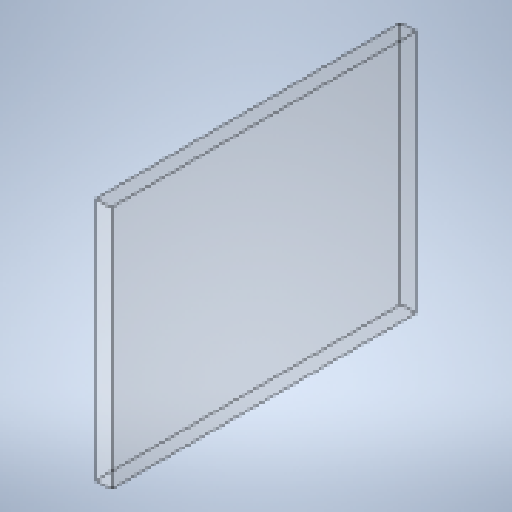
# Autodesk Inventor part: Cover
Saved by Autodesk Inventor 2023.2 (Build 272271000, 271)
## iProperties
Created: 2024-03-02
Part Number: Cover
Material: Polycarbonate, Clear
Document SubType Name: Modeling
Designer: Nathan Cai
Density: 1.2 g/cm^3
Appearance: Polycarbonate - Clear
Author: Nathan Cai
Autodesk Inventor part; units mm, degrees
ref_plane "YZ Plane" through (0, 0, 0) normal (1, 0, 0) x (0, 1, 0)
ref_plane "XZ Plane" through (0, 0, 0) normal (0, 1, 0) x (-1, 0, 0)
ref_plane "XY Plane" through (0, 0, 0) normal (0, 0, 1) x (1, 0, 0)
sketch "Sketch1" plane through (0, 0, 0) normal (1, 0, 0) x (0, 1, 0)
  line L0 (-22.225, -31.75) -> (22.225, -31.75)
  line L1 (22.225, -31.75) -> (22.225, 31.75)
  line L2 (22.225, 31.75) -> (-22.225, 31.75)
  line L3 (-22.225, 31.75) -> (-22.225, -31.75)
  line L4 (-22.225, -31.75) -> (22.225, 31.75) construction
  line L5 (22.225, -31.75) -> (-22.225, 31.75) construction
  point P0 (0, 0)
  dimension "d0" = 44.45
  dimension "d1" = 63.5
  constraints: 12 end point, 2 midpoint, 2 parallel, 1 horizontal, 1 perpendicular
  measures "d0" distance of L2.end L1.end
  measures "d1" distance of L1.end L0.end
extrude "Extrusion1" add sketch "Sketch1" along normal blind 3.175
body "Solid1"
